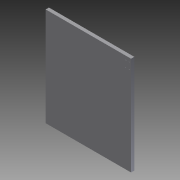
# Autodesk Inventor part: ajustableBase w mounting holes
Saved by Autodesk Inventor 2011 SP1 (Build 150282100, 282)
## iProperties
Created: 2013-01-18
Part Number: ajustableBase w mounting holes
Document SubType Name: Modeling
Designer: wes
Density: 1 g/cm^3
Author: wes
Autodesk Inventor part; units mm, degrees
ref_plane "YZ Plane" through (0, 0, 0) normal (1, 0, 0) x (0, 1, 0)
ref_plane "XZ Plane" through (0, 0, 0) normal (0, 1, 0) x (-1, 0, 0)
ref_plane "XY Plane" through (0, 0, 0) normal (0, 0, 1) x (1, 0, 0)
sketch "Sketch1" plane through (0, 0, 0) normal (0, 0, 1) x (1, 0, 0)
  line L0 (67.8531, 30.0133) -> (728.2531, 30.0133)
  line L1 (728.2531, 30.0133) -> (728.2531, -731.9867)
  line L2 (728.2531, -731.9867) -> (67.8531, -731.9867)
  line L3 (67.8531, -731.9867) -> (67.8531, 30.0133)
  point P0 (0, 0)
  dimension "d0" = 660.4
  dimension "d1" = 762
  constraints: 8 end point, 2 parallel, 1 horizontal, 1 perpendicular
  measures "d0" distance of L0.start L0.end
  measures "d1" distance of L2.end L0.start
extrude "Extrusion1" add sketch "Sketch1" against normal blind 25.4
sketch "Sketch2" plane through (0, 0, 0) normal (0, 0, 1) x (1, 0, 0)
  line L0 (728.2531, 30.0133) -> (728.2531, -731.9867) projected
  line L1 (687.6131, 1.7734) -> (713.0131, 1.7734)
  line L2 (713.0131, 1.7734) -> (713.0131, -49.0266)
  line L3 (713.0131, -49.0266) -> (687.6131, -49.0266)
  line L4 (687.6131, -49.0266) -> (687.6131, 1.7734)
  point P0 (0, 0)
  dimension "d11" = 25.4
  dimension "d12" = 50.8
  dimension "d13" = 15.24
  constraints: 8 end point, 4 coincident, 2 parallel, 1 horizontal, 1 perpendicular
  measures "d11" distance of L1.start L1.end
  measures "d12" distance of L3.end L1.start
  measures "d13" distance between parallel lines of L0 L2
hole "Hole1" at (687.6131, 1.7734, 0) at (713.0131, 1.7734, 0) at (713.0131, -49.0266, 0) at (687.6131, -49.0266, 0) direction (0, 0, -1) diameter 6.35 depth 50.8 tip angle 118
body "Solid1"
